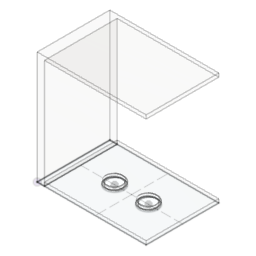
clamp base v1 (Autodesk Fusion 360 design; units mm, degrees)
Autodesk Fusion 360 part; units mm, degrees
sketch "Sketch1" plane through (0, 0, 0) normal (0, 0, 1) x (1, 0, 0)
  line L0 (0, 0) -> (76.2, 0)
  line L1 (76.2, 0) -> (76.2, 50.8)
  line L2 (76.2, 50.8) -> (0, 50.8)
  line L3 (0, 50.8) -> (0, 0)
  line L4 (0, 0) -> (5.08, 0)
  line L5 (5.08, 0) -> (5.08, 50.8)
  line L6 (5.08, 50.8) -> (0, 50.8)
  line L7 (0, 50.8) -> (0, 0)
  circle A0 centre (28.7867, 25.4) radius 6.35
  circle A1 centre (52.4933, 25.4) radius 6.35
  line L8 (52.4933, 25.4) -> (76.2, 25.4) construction
  line L9 (52.4933, 25.4) -> (28.7867, 25.4) construction
  line L10 (28.7867, 25.4) -> (5.08, 25.4) construction
  line L11 (40.64, 25.4) -> (40.64, 50.8) construction
  line L12 (40.64, 25.4) -> (40.64, 0) construction
  dimension "d1" = 76.2
  dimension "d2" = 50.8
  dimension "d3" = 5.08
  dimension "d12" = 12.7
  dimension "d13" = 12.7
  constraint horizontal L0
  constraint vertical L1
  constraint horizontal L2
  constraint vertical L3
  constraint coincident L0.start L3.end
  constraint horizontal L4
  constraint vertical L5
  constraint horizontal L6
  constraint vertical L7
  constraint equal L3 L5
  constraint coincident A1.centre L8.start
  constraint coincident L1 L8.end
  constraint perpendicular L1 L8
  constraint coincident A0.centre L9.end
  constraint parallel L8 L9
  constraint coincident L5 L10.end
  constraint perpendicular L5 L10
  constraint equal L8 L9
  constraint equal L9 L10
  constraint midpoint L9 L11.start
  constraint coincident L2 L11.end
  constraint perpendicular L2 L11
  constraint coincident L0 L12.end
  constraint perpendicular L0 L12
  constraint equal L11 L12
  measures "d1" distance of L0.start L0.end
  measures "d2" distance of L0.start L2.end
  measures "d3" distance of L0.start L4.end
  measures "d12" diameter of A0
  measures "d13" diameter of A1
extrude "Extrude1" add sketch "Sketch1" along normal blind 2.54 contours L0 L1 L2 L5 | A0 | A1 makes body 1
extrude "Extrude2" add sketch "Sketch1" along normal blind 76.2 separate body contours L0 L2 L3 L4 L5 L6 L7 makes body 2
sketch "Sketch2" plane through (0, 0, 76.2) normal (0, 0, 1) x (-1, 0, 0)
  line L0 (0, -50.8) -> (0, 0)
  line L1 (0, 0) -> (-5.08, 0)
  line L2 (-5.08, 0) -> (-5.08, -50.8)
  line L3 (-5.08, -50.8) -> (0, -50.8)
  line L4 (0, 0) -> (-76.2, 0)
  line L5 (-76.2, 0) -> (-76.2, -50.8)
  line L6 (-76.2, -50.8) -> (0, -50.8)
  line L7 (0, -50.8) -> (0, 0)
  dimension "d8" = 76.2
  dimension "d9" = 50.8
  constraint horizontal L4
  constraint vertical L5
  constraint horizontal L6
  constraint vertical L7
  constraint coincident L0.end L1.start
  measures "d8" distance of L0.end L4.end
  measures "d9" distance of L0.end L0.start
extrude "Extrude3" add sketch "Sketch2" along normal blind 2.54 bodies 2
extrude "Extrude4" cut sketch "Sketch1" along normal blind 12.7 contours A0 | A1 bodies 1
thread "Thread1" "ANSI Unified Screw Threads 0.5 1/2-12 UNS 3B" major diameter 12.7 minor diameter 10.5715 pitch 2.1167 angle 60 modelled right hand crest width 0.5847 on face at (35.1051, 26.0323, 1.6933) crest through (34.0724, 25.4, 0.5292) on bodies 1
thread "Thread2" "ANSI Unified Screw Threads 0.5 1/2-12 UNS 3B" major diameter 12.7 minor diameter 10.5715 pitch 2.1167 angle 60 modelled right hand crest width 0.5847 on face at (58.8354, 25.7165, 0.8467) crest through (57.7791, 25.4, 0.5292) on bodies 1
component "Component" placed x (1, 0, 0) y (0, 1, 0) z (0, 0, 1) at (0, 0, 0)
